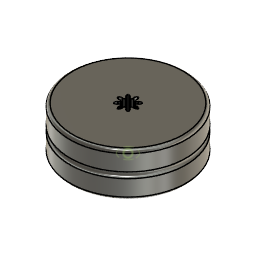
FlyWheel (Autodesk Fusion 360 design; units mm, degrees)
description: Spur Gear; Module: 0.7; Num Teeth: 8; Pressure Angle: 20.0; Backlash: 0.00 mm
Autodesk Fusion 360 part; units mm, degrees
sketch "Sketch1" plane through (0, 0, 0) normal (0, 0, 1) x (1, 0, 0)
  circle A0 centre (0, 0) radius 20
  dimension "d1" = 40
  constraint coincident A0.centre origin
  measures "d1" diameter of A0
extrude "Extrude1" add sketch "Sketch1" along normal blind 15 makes body 1
sketch "Sketch1 (2)" plane through (0, 0, 0) normal (0, 0, 1) x (1, 0, 0) in component "Spur Gear (8 teeth)"
  circle A0 centre (0, 0) radius 1.9092
extrude "Extrude1'" add sketch "Sketch1 (2)" along normal blind 20 separate body makes body 2 in component "Spur Gear (8 teeth)"
sketch "Sketch2" plane through (0, 0, 0) normal (0, 0, 1) x (1, 0, 0) in component "Spur Gear (8 teeth)"
  spline S0 degree 5 poles (2.5726, -0.5517) (2.5751, -0.5522) (2.5802, -0.5532) (2.5877, -0.5544) (2.5979, -0.5554) (2.6107, -0.556) (2.6236, -0.5561) (2.6366, -0.5558) (2.6496, -0.5554) (2.6626, -0.5548) (2.6757, -0.5541) (2.6888, -0.5532) (2.7019, -0.5521) (2.715, -0.5507) (2.7282, -0.549) (2.7415, -0.5471) (2.7547, -0.545) (2.768, -0.5427) (2.7812, -0.5402) (2.7945, -0.5376) (2.8079, -0.5348) (2.8212, -0.5319) (2.8345, -0.5287) (2.8479, -0.5254) (2.8612, -0.522) (2.8746, -0.5183) (2.888, -0.5145) (2.9014, -0.5106) (2.9148, -0.5065) (2.9282, -0.5022) (2.9416, -0.4978) (2.955, -0.4932) (2.9684, -0.4885) (2.9818, -0.4837) (2.9952, -0.4786) (3.0086, -0.4735) (3.022, -0.4682) (3.0354, -0.4628) (3.0488, -0.4572) (3.0621, -0.4515) (3.0755, -0.4456) (3.0889, -0.4396) (3.1022, -0.4335) (3.1156, -0.4272) (3.1289, -0.4208) (3.1423, -0.4143) (3.1556, -0.4076) (3.1689, -0.4008) (3.1822, -0.3938) (3.1954, -0.3868) (3.2087, -0.3796) (3.222, -0.3722) (3.2352, -0.3648) (3.2484, -0.3572) (3.2616, -0.3495) (3.2747, -0.3416) (3.2879, -0.3337) (3.301, -0.3256) (3.3141, -0.3173) (3.3272, -0.309) (3.3403, -0.3005) (3.3533, -0.2919) (3.3663, -0.2832) (3.3793, -0.2744) (3.3923, -0.2654) (3.4052, -0.2563) (3.4181, -0.2471) (3.431, -0.2378) (3.4438, -0.2283) (3.4566, -0.2188) (3.4694, -0.2091) (3.4796, -0.2013) (3.4872, -0.1953) (3.4923, -0.1913) (3.4949, -0.1893) knots 0 0 0 0 0 0 0.01428571 0.02857143 0.04285714 0.05714286 0.07142857 0.08571429 0.1 0.11428571 0.12857143 0.14285714 0.15714286 0.17142857 0.18571429 0.2 0.21428571 0.22857143 0.24285714 0.25714286 0.27142857 0.28571429 0.3 0.31428571 0.32857143 0.34285714 0.35714286 0.37142857 0.38571429 0.4 0.41428571 0.42857143 0.44285714 0.45714286 0.47142857 0.48571429 0.5 0.51428571 0.52857143 0.54285714 0.55714286 0.57142857 0.58571429 0.6 0.61428571 0.62857143 0.64285714 0.65714286 0.67142857 0.68571429 0.7 0.71428571 0.72857143 0.74285714 0.75714286 0.77142857 0.78571429 0.8 0.81428571 0.82857143 0.84285714 0.85714286 0.87142857 0.88571429 0.9 0.91428571 0.92857143 0.94285714 0.95714286 0.97142857 0.98571429 1 1 1 1 1 1
  spline S1 degree 5 poles (2.5726, 0.5517) (2.5751, 0.5522) (2.5802, 0.5532) (2.5877, 0.5544) (2.5979, 0.5554) (2.6107, 0.556) (2.6236, 0.5561) (2.6366, 0.5558) (2.6496, 0.5554) (2.6626, 0.5548) (2.6757, 0.5541) (2.6888, 0.5532) (2.7019, 0.5521) (2.715, 0.5507) (2.7282, 0.549) (2.7415, 0.5471) (2.7547, 0.545) (2.768, 0.5427) (2.7812, 0.5402) (2.7945, 0.5376) (2.8079, 0.5348) (2.8212, 0.5319) (2.8345, 0.5287) (2.8479, 0.5254) (2.8612, 0.522) (2.8746, 0.5183) (2.888, 0.5145) (2.9014, 0.5106) (2.9148, 0.5065) (2.9282, 0.5022) (2.9416, 0.4978) (2.955, 0.4932) (2.9684, 0.4885) (2.9818, 0.4837) (2.9952, 0.4786) (3.0086, 0.4735) (3.022, 0.4682) (3.0354, 0.4628) (3.0488, 0.4572) (3.0621, 0.4515) (3.0755, 0.4456) (3.0889, 0.4396) (3.1022, 0.4335) (3.1156, 0.4272) (3.1289, 0.4208) (3.1423, 0.4143) (3.1556, 0.4076) (3.1689, 0.4008) (3.1822, 0.3938) (3.1954, 0.3868) (3.2087, 0.3796) (3.222, 0.3722) (3.2352, 0.3648) (3.2484, 0.3572) (3.2616, 0.3495) (3.2747, 0.3416) (3.2879, 0.3337) (3.301, 0.3256) (3.3141, 0.3173) (3.3272, 0.309) (3.3403, 0.3005) (3.3533, 0.2919) (3.3663, 0.2832) (3.3793, 0.2744) (3.3923, 0.2654) (3.4052, 0.2563) (3.4181, 0.2471) (3.431, 0.2378) (3.4438, 0.2283) (3.4566, 0.2188) (3.4694, 0.2091) (3.4796, 0.2013) (3.4872, 0.1953) (3.4923, 0.1913) (3.4949, 0.1893) knots 0 0 0 0 0 0 0.01428571 0.02857143 0.04285714 0.05714286 0.07142857 0.08571429 0.1 0.11428571 0.12857143 0.14285714 0.15714286 0.17142857 0.18571429 0.2 0.21428571 0.22857143 0.24285714 0.25714286 0.27142857 0.28571429 0.3 0.31428571 0.32857143 0.34285714 0.35714286 0.37142857 0.38571429 0.4 0.41428571 0.42857143 0.44285714 0.45714286 0.47142857 0.48571429 0.5 0.51428571 0.52857143 0.54285714 0.55714286 0.57142857 0.58571429 0.6 0.61428571 0.62857143 0.64285714 0.65714286 0.67142857 0.68571429 0.7 0.71428571 0.72857143 0.74285714 0.75714286 0.77142857 0.78571429 0.8 0.81428571 0.82857143 0.84285714 0.85714286 0.87142857 0.88571429 0.9 0.91428571 0.92857143 0.94285714 0.95714286 0.97142857 0.98571429 1 1 1 1 1 1
  arc A0 (3.4949, -0.1893) -> (3.4949, 0.1893) centre (0, 0) ccw
  line L0 (1.857, -0.4003) -> (2.5726, -0.5517)
  line L1 (1.857, 0.4003) -> (2.5726, 0.5517)
  line L2 (1.857, -0.4003) -> (1.857, 0.4003)
  point P0 (2.6352, -0.5558)
  point P1 (2.6994, -0.5522)
  point P2 (2.7644, -0.5433)
  point P3 (2.8302, -0.5297)
  point P4 (2.8965, -0.512)
  point P5 (2.9632, -0.4903)
  point P6 (3.0301, -0.4649)
  point P7 (3.0971, -0.4358)
  point P8 (3.1641, -0.4032)
  point P9 (3.231, -0.3671)
  point P10 (3.2976, -0.3277)
  point P11 (3.3638, -0.2849)
  point P12 (3.4296, -0.2387)
  point P13 (2.6352, 0.5558)
  point P14 (2.6994, 0.5522)
  point P15 (2.7644, 0.5433)
  point P16 (2.8302, 0.5297)
  point P17 (2.8965, 0.512)
  point P18 (2.9632, 0.4903)
  point P19 (3.0301, 0.4649)
  point P20 (3.0971, 0.4358)
  point P21 (3.1641, 0.4032)
  point P22 (3.231, 0.3671)
  point P23 (3.2976, 0.3277)
  point P24 (3.3638, 0.2849)
  point P25 (3.4296, 0.2387)
extrude "Extrude2" add sketch "Sketch2" along normal blind 20 bodies 2 in component "Spur Gear (8 teeth)"
fillet "Fillet1" radius 0.4 2 edges at (1.8663, -0.4023, 10) (1.8663, 0.4023, 10) on bodies 2 in component "Spur Gear (8 teeth)"
pattern_circular "C-Pattern1" count 8 over 360 about axis through (0, 0, 0) along (0, 0, 1) of "Extrude2", "Fillet1" in component "Spur Gear (8 teeth)"
sketch "Sketch3" plane through (0, 0, 0) normal (0, 0, 1) x (1, 0, 0) in component "Spur Gear (8 teeth)"
  circle A0 centre (0, 0) radius 2.8 construction
combine "Combine4" operation cut target body 1 tool bodies 2
sketch "Sketch2 (2)" plane through (0, 0, 0) normal (0, 1, 0) x (1, 0, 0)
  line L0 (-20, -15) -> (20, -15)
  line L1 (-20, 0) -> (20, 0)
  line L2 (20, -15) -> (20, 0) construction
  circle A0 centre (20, -7.5) radius 1
  dimension "d50" = 2
  constraint coincident L0.end L2.start
  constraint coincident L1.end L2.end
  constraint midpoint L2 A0.centre
  measures "d50" diameter of A0
revolve "Revolve1" cut sketch "Sketch2 (2)" angle 360 about axis through (0, 0, -7.5) along (0, 0, 1) bodies 1
fillet "Fillet3" radius 1 2 edges at (-18.6465, -7.2323, 15) (-18.6465, -7.2323, 0) on bodies 1
component "Spur Gear (8 teeth)" placed x (1, 0, 0) y (0, 1, 0) z (0, 0, 1) at (0, 0, 0)
